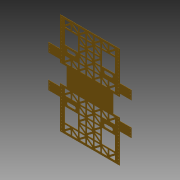
# Autodesk Inventor part: Top Plate
Saved by Autodesk Inventor 2014 SP1 (Build 180222100, 222)
## iProperties
Created: 2014-01-19
Part Number: Top Plate
Material: Aluminum 6061
Document SubType Name: Sheet Metal
Designer: Nick
Density: 2.71 g/cm^3
Appearance: Brass - Satin
Mass: 1865.48 g
Surface Area: 6483.38 cm^2
Volume: 688.368 cm^3
Sheet Metal Rule: Default
Author: Nick
Autodesk Inventor part; units mm, degrees
(part 1 of 3)
ref_plane "YZ Plane" through (0, 0, 0) normal (1, 0, 0) x (0, 1, 0)
ref_plane "XZ Plane" through (0, 0, 0) normal (0, 1, 0) x (-1, 0, 0)
ref_plane "XY Plane" through (0, 0, 0) normal (0, 0, 1) x (1, 0, 0)
sketch "Sketch1" plane through (0, 0, 0) normal (0, 0, 1) x (1, 0, 0)
  line L0 (-228.6, 152.4) -> (-228.6, 406.4)
  line L1 (-228.6, 406.4) -> (279.4, 406.4)
  line L2 (279.4, 406.4) -> (279.4, 152.4)
  line L3 (279.4, 152.4) -> (381, 152.4)
  line L4 (381, 152.4) -> (381, 76.2)
  line L5 (381, 76.2) -> (279.4, 76.2)
  line L6 (279.4, 76.2) -> (279.4, -127)
  line L7 (279.4, -127) -> (381, -127)
  line L8 (381, -127) -> (381, -203.2)
  line L9 (381, -203.2) -> (279.4, -203.2)
  line L10 (279.4, -203.2) -> (279.4, -457.2)
  line L11 (279.4, -457.2) -> (-228.6, -457.2)
  line L12 (-228.6, -457.2) -> (-228.6, -203.2)
  line L13 (-228.6, -203.2) -> (-330.2, -203.2)
  line L14 (-330.2, -203.2) -> (-330.2, -127)
  line L15 (-330.2, -127) -> (-228.6, -127)
  line L16 (-228.6, -127) -> (-228.6, 76.2)
  line L17 (-228.6, 76.2) -> (-330.2, 76.2)
  line L18 (-330.2, 76.2) -> (-330.2, 152.4)
  line L19 (-330.2, 152.4) -> (-228.6, 152.4)
  point P0 (0, 0)
  point P1 (279.4, 279.4)
  point P2 (279.4, -25.4)
  point P3 (279.4, -330.2)
  point P4 (381, -165.1)
  point P5 (381, 114.3)
  point P6 (-228.6, 279.4)
  point P7 (-228.6, -25.4)
  point P8 (-228.6, -330.2)
  point P9 (-330.2, -165.1)
  point P10 (-330.2, 114.3)
  point P11 (330.2, 76.2)
  point P12 (-279.4, 76.2)
  point P13 (-279.4, 152.4)
  point P14 (330.2, 152.4)
  point P15 (330.2, -127)
  point P16 (-279.4, -127)
  point P17 (-279.4, -203.2)
  point P18 (330.2, -203.2)
  dimension "d0" = 101.6
  dimension "d1" = 508
  dimension "d2" = 254
  dimension "d3" = 76.2
  dimension "d4" = 203.2
  dimension "d96" = 457.2
  dimension "d97" = 279.4
  constraints: 40 end point, 18 midpoint, 9 perpendicular, 6 horizontal, 6 vertical alignment, 5 collinear, 4 horizontal alignment, 2 parallel, 1 vertical
  measures "d0" distance from line of point (381, 114.3) L2
  measures "d1" distance of L0.end L1.end
  measures "d2" distance of L1.end L2.end
  measures "d3" distance of L3.end L4.end
  measures "d4" distance of L5.end L6.end
  measures "d96" distance from line of point (0, 0) L11
  measures "d97" distance from line of L6 point (0, 0)
extrude "Extrusion1" add sketch "Sketch1" along normal blind 2.286
sketch "Sketch2" plane through (0, 0, 2.286) normal (0, 0, 1) x (1, 0, 0)
  line L0 (-228.6, 406.4) -> (279.4, 406.4) projected
  line L1 (-228.6, 152.4) -> (-228.6, 406.4) projected
  line L2 (-330.2, 76.2) -> (-330.2, 152.4) projected
  line L3 (381, 152.4) -> (381, 76.2) projected
  line L4 (279.4, 406.4) -> (279.4, 152.4) projected
  point P0 (0, 0)
  point P1 (-215.9, 393.7)
  point P2 (266.7, 393.7)
  point P3 (-215.9, 368.3)
  point P4 (266.7, 368.3)
  point P5 (-215.9, 342.9)
  point P6 (266.7, 342.9)
  point P7 (-215.9, 317.5)
  point P8 (266.7, 317.5)
  point P9 (-215.9, 292.1)
  point P10 (266.7, 292.1)
  point P11 (-215.9, 266.7)
  point P12 (266.7, 266.7)
  point P13 (-215.9, 241.3)
  point P14 (266.7, 241.3)
  point P15 (-215.9, 215.9)
  point P16 (266.7, 215.9)
  point P17 (-215.9, 190.5)
  point P18 (266.7, 190.5)
  point P19 (-215.9, 165.1)
  point P20 (266.7, 165.1)
  point P21 (-215.9, 139.7)
  point P22 (266.7, 139.7)
  point P23 (-215.9, 114.3)
  point P24 (266.7, 114.3)
  point P25 (-215.9, 88.9)
  point P26 (266.7, 88.9)
  point P27 (-215.9, 63.5)
  point P28 (266.7, 63.5)
  point P29 (-215.9, 38.1)
  point P30 (266.7, 38.1)
  point P31 (-215.9, 12.7)
  point P32 (266.7, 12.7)
  point P33 (-215.9, -12.7)
  point P34 (266.7, -12.7)
  point P35 (-215.9, -38.1)
  point P36 (266.7, -38.1)
  point P37 (-215.9, -63.5)
  point P38 (266.7, -63.5)
  point P39 (-215.9, -88.9)
  point P40 (266.7, -88.9)
  point P41 (-215.9, -114.3)
  point P42 (266.7, -114.3)
  point P43 (-215.9, -139.7)
  point P44 (266.7, -139.7)
  point P45 (-215.9, -165.1)
  point P46 (266.7, -165.1)
  point P47 (-215.9, -190.5)
  point P48 (266.7, -190.5)
  point P49 (-215.9, -215.9)
  point P50 (266.7, -215.9)
  point P51 (-215.9, -241.3)
  point P52 (266.7, -241.3)
  point P53 (-215.9, -266.7)
  point P54 (266.7, -266.7)
  point P55 (-215.9, -292.1)
  point P56 (266.7, -292.1)
  point P57 (-215.9, -317.5)
  point P58 (266.7, -317.5)
  point P59 (-215.9, -342.9)
  point P60 (266.7, -342.9)
  point P61 (-215.9, -368.3)
  point P62 (266.7, -368.3)
  point P63 (-215.9, -393.7)
  point P64 (266.7, -393.7)
  point P65 (-215.9, -419.1)
  point P66 (266.7, -419.1)
  point P67 (-215.9, -444.5)
  point P68 (266.7, -444.5)
  point P69 (-317.5, 139.7)
  point P70 (-317.5, 114.3)
  point P71 (-317.5, 88.9)
  point P72 (-317.5, -139.7)
  point P73 (-317.5, -165.1)
  point P74 (-317.5, -190.5)
  point P75 (368.3, -139.7)
  point P76 (368.3, -165.1)
  point P77 (368.3, -190.5)
  point P78 (368.3, 139.7)
  point P79 (368.3, 114.3)
  point P80 (368.3, 88.9)
  dimension "d7" = 12.7
  dimension "d8" = 12.7
  dimension "d9" = 12.7
  dimension "d10" = 12.7
  dimension "d13" = 25.4
  dimension "d18" = 12.7
  dimension "d19" = 12.7
  constraints: 12 horizontal alignment, 10 vertical alignment, 1 vertical, 66 other
  measures "d7" distance from line of point (-215.9, 393.7) L1
  measures "d8" distance from line of L0 point (-215.9, 393.7)
  measures "d9" distance from line of L0 point (266.7, 393.7)
  measures "d10" distance from line of L4 point (266.7, 393.7)
  measures "d13" distance of point (-215.9, 393.7) point (-215.9, 368.3)
  measures "d18" distance from line of L3 point (368.3, 114.3)
  measures "d19" distance from line of L2 point (-317.5, 139.7)
hole "Hole1" at (-215.9, 393.7, 2.286) at (266.7, 393.7, 2.286) at (-215.9, 368.3, 2.286) at (266.7, 368.3, 2.286) at (-215.9, 342.9, 2.286) at (266.7, 342.9, 2.286) at (-215.9, 317.5, 2.286) at (266.7, 317.5, 2.286) at (-215.9, 292.1, 2.286) at (266.7, 292.1, 2.286) at (-215.9, 266.7, 2.286) at (266.7, 266.7, 2.286) at (-215.9, 241.3, 2.286) at (266.7, 241.3, 2.286) at (-215.9, 215.9, 2.286) at (266.7, 215.9, 2.286) at (-215.9, 190.5, 2.286) at (266.7, 190.5, 2.286) at (-215.9, 165.1, 2.286) at (266.7, 165.1, 2.286) at (-215.9, 139.7, 2.286) at (266.7, 139.7, 2.286) at (-215.9, 114.3, 2.286) at (266.7, 114.3, 2.286) at (-215.9, 88.9, 2.286) at (266.7, 88.9, 2.286) at (-215.9, 63.5, 2.286) at (266.7, 63.5, 2.286) at (-215.9, 38.1, 2.286) at (266.7, 38.1, 2.286) at (-215.9, 12.7, 2.286) at (266.7, 12.7, 2.286) at (-215.9, -12.7, 2.286) at (266.7, -12.7, 2.286) at (-215.9, -38.1, 2.286) at (266.7, -38.1, 2.286) at (-215.9, -63.5, 2.286) at (266.7, -63.5, 2.286) at (-215.9, -88.9, 2.286) at (266.7, -88.9, 2.286) at (-215.9, -114.3, 2.286) at (266.7, -114.3, 2.286) at (-215.9, -139.7, 2.286) at (266.7, -139.7, 2.286) at (-215.9, -165.1, 2.286) at (266.7, -165.1, 2.286) at (-215.9, -190.5, 2.286) at (266.7, -190.5, 2.286) at (-215.9, -215.9, 2.286) at (266.7, -215.9, 2.286) direction (0, 0, -1) diameter 6.7564 end through all and at (-215.9, -241.3, 2.286) (266.7, -241.3, 2.286) (-215.9, -266.7, 2.286) (266.7, -266.7, 2.286) (-215.9, -292.1, 2.286) (266.7, -292.1, 2.286) (-215.9, -317.5, 2.286) (266.7, -317.5, 2.286) (-215.9, -342.9, 2.286) (266.7, -342.9, 2.286) (-215.9, -368.3, 2.286) (266.7, -368.3, 2.286) (-215.9, -393.7, 2.286) (266.7, -393.7, 2.286) (-215.9, -419.1, 2.286) (266.7, -419.1, 2.286) (-215.9, -444.5, 2.286) (266.7, -444.5, 2.286) (-317.5, 139.7, 2.286) (-317.5, 114.3, 2.286) (-317.5, 88.9, 2.286) (-317.5, -139.7, 2.286) (-317.5, -165.1, 2.286) (-317.5, -190.5, 2.286) (368.3, -139.7, 2.286) (368.3, -165.1, 2.286) (368.3, -190.5, 2.286) (368.3, 139.7, 2.286) (368.3, 114.3, 2.286) (368.3, 88.9, 2.286)
sketch "Sketch4" plane through (0, 0, 2.286) normal (0, 0, 1) x (1, 0, 0)
  circle A0 centre (266.7, -88.9) radius 3.3782 projected
  circle A1 centre (-215.9, -88.9) radius 3.3782 projected
  circle A2 centre (266.7, -63.5) radius 3.3782 projected
  circle A3 centre (-215.9, -63.5) radius 3.3782 projected
  circle A4 centre (266.7, -38.1) radius 3.3782 projected
  circle A5 centre (-215.9, -38.1) radius 3.3782 projected
  circle A6 centre (266.7, -12.7) radius 3.3782 projected
  circle A7 centre (-215.9, -12.7) radius 3.3782 projected
  circle A8 centre (266.7, 12.7) radius 3.3782 projected
  circle A9 centre (-215.9, 12.7) radius 3.3782 projected
  circle A10 centre (266.7, 38.1) radius 3.3782 projected
  circle A11 centre (-215.9, 38.1) radius 3.3782 projected
  line L0 (-228.6, 76.2) -> (-330.2, 76.2) projected
  line L1 (-228.6, -127) -> (-228.6, 76.2) projected
  line L2 (279.4, 76.2) -> (279.4, -127) projected
  line L3 (381, 76.2) -> (279.4, 76.2) projected
  line L4 (-228.6, -101.6) -> (-171.45, -101.6)
  line L5 (-171.45, -101.6) -> (-171.45, 50.8)
  line L6 (-171.45, 50.8) -> (-228.6, 50.8)
  line L7 (-228.6, 50.8) -> (-228.6, -101.6)
  line L8 (279.4, -101.6) -> (222.25, -101.6)
  line L9 (222.25, -101.6) -> (222.25, 50.8)
  line L10 (222.25, 50.8) -> (279.4, 50.8)
  line L11 (279.4, 50.8) -> (279.4, -101.6)
  point P0 (0, 0)
  dimension "d27" = 152.4
  dimension "d28" = 57.15
  dimension "d29" = 57.15
  dimension "d30" = 152.4
  dimension "d31" = 25.4
  dimension "d32" = 25.4
  constraints: 16 end point, 4 parallel, 2 horizontal, 2 perpendicular, 2 point on line
  measures "d27" distance of L8.end L9.end
  measures "d28" distance of L9.end L10.end
  measures "d29" distance of L5.end L6.end
  measures "d30" distance of L4.end L5.end
  measures "d31" distance between parallel lines of L0 L6
  measures "d32" distance between parallel lines of L3 L10
extrude "Extrusion2" cut sketch "Sketch4" against normal through all
sketch "Sketch6" plane through (0, 0, 2.286) normal (0, 0, 1) x (1, 0, 0)
  line L0 (-171.45, -101.6) -> (-228.6, -101.6) projected
  line L1 (-228.6, -127) -> (-228.6, -101.6) projected
  line L2 (-330.2, -127) -> (-228.6, -127) projected
  line L3 (-330.2, -203.2) -> (-330.2, -127) projected
  line L4 (-228.6, -203.2) -> (-330.2, -203.2) projected
  line L5 (-228.6, -457.2) -> (-228.6, -203.2) projected
  line L6 (279.4, -457.2) -> (-228.6, -457.2) projected
  line L7 (279.4, -203.2) -> (279.4, -457.2) projected
  line L8 (381, -203.2) -> (279.4, -203.2) projected
  line L9 (381, -127) -> (381, -203.2) projected
  line L10 (279.4, -127) -> (381, -127) projected
  line L11 (279.4, -101.6) -> (279.4, -127) projected
  line L12 (279.4, -101.6) -> (222.25, -101.6) projected
  line L13 (222.25, -101.6) -> (222.25, 50.8) projected
  line L14 (279.4, 76.2) -> (279.4, 50.8) projected
  line L15 (381, 76.2) -> (279.4, 76.2) projected
  line L16 (381, 152.4) -> (381, 76.2) projected
  line L17 (279.4, 152.4) -> (381, 152.4) projected
  line L18 (279.4, 406.4) -> (279.4, 152.4) projected
  line L19 (-228.6, 406.4) -> (279.4, 406.4) projected
  line L20 (-228.6, 152.4) -> (-228.6, 406.4) projected
  line L21 (-330.2, 152.4) -> (-228.6, 152.4) projected
  line L22 (-330.2, 76.2) -> (-330.2, 152.4) projected
  line L23 (-228.6, 76.2) -> (-330.2, 76.2) projected
  line L24 (-228.6, 50.8) -> (-228.6, 76.2) projected
  line L25 (-171.45, 50.8) -> (-171.45, -101.6) projected
  circle A0 centre (368.3, 88.9) radius 3.3782 projected
  circle A1 centre (368.3, 114.3) radius 3.3782 projected
  circle A2 centre (368.3, 139.7) radius 3.3782 projected
  circle A3 centre (368.3, -190.5) radius 3.3782 projected
  circle A4 centre (368.3, -165.1) radius 3.3782 projected
  circle A5 centre (368.3, -139.7) radius 3.3782 projected
  circle A6 centre (-317.5, -190.5) radius 3.3782 projected
  circle A7 centre (-317.5, -165.1) radius 3.3782 projected
  circle A8 centre (-317.5, -139.7) radius 3.3782 projected
  circle A9 centre (-317.5, 88.9) radius 3.3782 projected
  circle A10 centre (-317.5, 114.3) radius 3.3782 projected
  circle A11 centre (-317.5, 139.7) radius 3.3782 projected
  circle A12 centre (266.7, -444.5) radius 3.3782 projected
  circle A13 centre (-215.9, -444.5) radius 3.3782 projected
  circle A14 centre (266.7, -419.1) radius 3.3782 projected
  circle A15 centre (-215.9, -419.1) radius 3.3782 projected
  circle A16 centre (266.7, -393.7) radius 3.3782 projected
  circle A17 centre (-215.9, -393.7) radius 3.3782 projected
  circle A18 centre (266.7, -368.3) radius 3.3782 projected
  circle A19 centre (-215.9, -368.3) radius 3.3782 projected
  circle A20 centre (266.7, -342.9) radius 3.3782 projected
  circle A21 centre (-215.9, -342.9) radius 3.3782 projected
  circle A22 centre (266.7, -317.5) radius 3.3782 projected
  circle A23 centre (-215.9, -317.5) radius 3.3782 projected
  circle A24 centre (266.7, -292.1) radius 3.3782 projected
  circle A25 centre (-215.9, -292.1) radius 3.3782 projected
  circle A26 centre (266.7, -266.7) radius 3.3782 projected
  circle A27 centre (-215.9, -266.7) radius 3.3782 projected
  circle A28 centre (266.7, -241.3) radius 3.3782 projected
  circle A29 centre (-215.9, -241.3) radius 3.3782 projected
  circle A30 centre (266.7, -215.9) radius 3.3782 projected
  circle A31 centre (-215.9, -215.9) radius 3.3782 projected
  circle A32 centre (266.7, -190.5) radius 3.3782 projected
  circle A33 centre (-215.9, -190.5) radius 3.3782 projected
  circle A34 centre (266.7, -165.1) radius 3.3782 projected
  circle A35 centre (-215.9, -165.1) radius 3.3782 projected
  circle A36 centre (266.7, -139.7) radius 3.3782 projected
  circle A37 centre (-215.9, -139.7) radius 3.3782 projected
  circle A38 centre (266.7, -114.3) radius 3.3782 projected
  circle A39 centre (-215.9, -114.3) radius 3.3782 projected
  line L26 (-190.5, 385.7625) -> (-190.5, 357.1875)
  line L27 (-185.42, 354.6475) -> (-147.32, 383.2225)
  line L28 (-149.225, 388.9375) -> (-187.325, 388.9375)
  line L29 (-182.88, 340.6775) -> (-144.78, 369.2525)
  line L30 (-139.7, 366.7125) -> (-139.7, 338.1375)
  line L31 (-142.875, 334.9625) -> (-180.975, 334.9625)
  arc A40 (-190.5, 357.1875) -> (-185.42, 354.6475) centre (-187.325, 357.1875) ccw
  arc A41 (-187.325, 388.9375) -> (-190.5, 385.7625) centre (-187.325, 385.7625) ccw
  arc A42 (-147.32, 383.2225) -> (-149.225, 388.9375) centre (-149.225, 385.7625) ccw
  arc A43 (-139.7, 366.7125) -> (-144.78, 369.2525) centre (-142.875, 366.7125) ccw
  arc A44 (-142.875, 334.9625) -> (-139.7, 338.1375) centre (-142.875, 338.1375) ccw
  arc A45 (-182.88, 340.6775) -> (-180.975, 334.9625) centre (-180.975, 338.1375) ccw
  line L32 (-133.35, 390.3218) -> (-133.35, 314.1218) construction
  line L33 (-76.2, 385.7625) -> (-76.2, 357.1875)
  line L34 (-81.28, 354.6475) -> (-119.38, 383.2225)
  line L35 (-117.475, 388.9375) -> (-79.375, 388.9375)
  line L36 (-83.82, 340.6775) -> (-121.92, 369.2525)
  line L37 (-127, 366.7125) -> (-127, 338.1375)
  line L38 (-123.825, 334.9625) -> (-85.725, 334.9625)
  arc A46 (-81.28, 354.6475) -> (-76.2, 357.1875) centre (-79.375, 357.1875) ccw
  arc A47 (-76.2, 385.7625) -> (-79.375, 388.9375) centre (-79.375, 385.7625) ccw
  arc A48 (-117.475, 388.9375) -> (-119.38, 383.2225) centre (-117.475, 385.7625) ccw
  arc A49 (-121.92, 369.2525) -> (-127, 366.7125) centre (-123.825, 366.7125) ccw
  arc A50 (-127, 338.1375) -> (-123.825, 334.9625) centre (-123.825, 338.1375) ccw
  arc A51 (-85.725, 334.9625) -> (-83.82, 340.6775) centre (-85.725, 338.1375) ccw
  line L39 (-192.1848, 328.6125) -> (-47.7209, 328.6125) construction
  line L40 (-190.5, 271.4625) -> (-190.5, 300.0375)
  line L41 (-185.42, 302.5775) -> (-147.32, 274.0025)
  line L42 (-149.225, 268.2875) -> (-187.325, 268.2875)
  line L43 (-182.88, 316.5475) -> (-144.78, 287.9725)
  line L44 (-139.7, 290.5125) -> (-139.7, 319.0875)
  line L45 (-142.875, 322.2625) -> (-180.975, 322.2625)
  arc A52 (-185.42, 302.5775) -> (-190.5, 300.0375) centre (-187.325, 300.0375) ccw
  arc A53 (-190.5, 271.4625) -> (-187.325, 268.2875) centre (-187.325, 271.4625) ccw
  arc A54 (-149.225, 268.2875) -> (-147.32, 274.0025) centre (-149.225, 271.4625) ccw
  arc A55 (-144.78, 287.9725) -> (-139.7, 290.5125) centre (-142.875, 290.5125) ccw
  arc A56 (-139.7, 319.0875) -> (-142.875, 322.2625) centre (-142.875, 319.0875) ccw
  arc A57 (-180.975, 322.2625) -> (-182.88, 316.5475) centre (-180.975, 319.0875) ccw
  line L46 (-127, 290.5125) -> (-127, 319.0875)
  arc A58 (-127, 290.5125) -> (-121.92, 287.9725) centre (-123.825, 290.5125) ccw
  arc A59 (-119.38, 274.0025) -> (-117.475, 268.2875) centre (-117.475, 271.4625) ccw
  line L47 (-76.2, 271.4625) -> (-76.2, 300.0375)
  arc A60 (-79.375, 268.2875) -> (-76.2, 271.4625) centre (-79.375, 271.4625) ccw
  line L48 (-117.475, 268.2875) -> (-79.375, 268.2875)
  arc A61 (-83.82, 316.5475) -> (-85.725, 322.2625) centre (-85.725, 319.0875) ccw
  line L49 (-81.28, 302.5775) -> (-119.38, 274.0025)
  line L50 (-83.82, 316.5475) -> (-121.92, 287.9725)
  line L51 (-123.825, 322.2625) -> (-85.725, 322.2625)
  arc A62 (-76.2, 300.0375) -> (-81.28, 302.5775) centre (-79.375, 300.0375) ccw
  arc A63 (-123.825, 322.2625) -> (-127, 319.0875) centre (-123.825, 319.0875) ccw
  line L52 (-63.5, 385.7625) -> (-63.5, 357.1875)
  line L53 (-58.42, 354.6475) -> (-20.32, 383.2225)
  line L54 (-22.225, 388.9375) -> (-60.325, 388.9375)
  line L55 (-55.88, 340.6775) -> (-17.78, 369.2525)
  line L56 (-12.7, 366.7125) -> (-12.7, 338.1375)
  line L57 (-15.875, 334.9625) -> (-53.975, 334.9625)
  arc A64 (-63.5, 357.1875) -> (-58.42, 354.6475) centre (-60.325, 357.1875) ccw
  arc A65 (-60.325, 388.9375) -> (-63.5, 385.7625) centre (-60.325, 385.7625) ccw
  arc A66 (-20.32, 383.2225) -> (-22.225, 388.9375) centre (-22.225, 385.7625) ccw
  arc A67 (-12.7, 366.7125) -> (-17.78, 369.2525) centre (-15.875, 366.7125) ccw
  arc A68 (-15.875, 334.9625) -> (-12.7, 338.1375) centre (-15.875, 338.1375) ccw
  arc A69 (-55.88, 340.6775) -> (-53.975, 334.9625) centre (-53.975, 338.1375) ccw
  line L58 (-6.35, 391.9093) -> (-6.35, 315.7093) construction
  line L59 (0, 366.7125) -> (0, 338.1375)
  arc A70 (5.08, 369.2525) -> (0, 366.7125) centre (3.175, 366.7125) ccw
  arc A71 (9.525, 388.9375) -> (7.62, 383.2225) centre (9.525, 385.7625) ccw
  line L60 (50.8, 385.7625) -> (50.8, 357.1875)
  arc A72 (50.8, 385.7625) -> (47.625, 388.9375) centre (47.625, 385.7625) ccw
  line L61 (9.525, 388.9375) -> (47.625, 388.9375)
  arc A73 (41.275, 334.9625) -> (43.18, 340.6775) centre (41.275, 338.1375) ccw
  line L62 (45.72, 354.6475) -> (7.62, 383.2225)
  line L63 (43.18, 340.6775) -> (5.08, 369.2525)
  line L64 (3.175, 334.9625) -> (41.275, 334.9625)
  arc A74 (45.72, 354.6475) -> (50.8, 357.1875) centre (47.625, 357.1875) ccw
  arc A75 (0, 338.1375) -> (3.175, 334.9625) centre (3.175, 338.1375) ccw
  line L65 (-190.5973, 328.6125) -> (-46.1334, 328.6125) construction
  line L66 (0, 290.5125) -> (0, 319.0875)
  arc A76 (-53.975, 322.2625) -> (-55.88, 316.5475) centre (-53.975, 319.0875) ccw
  line L67 (-15.875, 322.2625) -> (-53.975, 322.2625)
  arc A77 (-12.7, 319.0875) -> (-15.875, 322.2625) centre (-15.875, 319.0875) ccw
  line L68 (-63.5, 271.4625) -> (-63.5, 300.0375)
  line L69 (-55.88, 316.5475) -> (-17.78, 287.9725)
  line L70 (-12.7, 290.5125) -> (-12.7, 319.0875)
  line L71 (-58.42, 302.5775) -> (-20.32, 274.0025)
  arc A78 (-22.225, 268.2875) -> (-20.32, 274.0025) centre (-22.225, 271.4625) ccw
  line L72 (-22.225, 268.2875) -> (-60.325, 268.2875)
  arc A79 (-17.78, 287.9725) -> (-12.7, 290.5125) centre (-15.875, 290.5125) ccw
  line L73 (50.8, 271.4625) -> (50.8, 300.0375)
  arc A80 (-58.42, 302.5775) -> (-63.5, 300.0375) centre (-60.325, 300.0375) ccw
  arc A81 (3.175, 322.2625) -> (0, 319.0875) centre (3.175, 319.0875) ccw
  arc A82 (0, 290.5125) -> (5.08, 287.9725) centre (3.175, 290.5125) ccw
  arc A83 (-63.5, 271.4625) -> (-60.325, 268.2875) centre (-60.325, 271.4625) ccw
  line L74 (3.175, 322.2625) -> (41.275, 322.2625)
  line L75 (43.18, 316.5475) -> (5.08, 287.9725)
  arc A84 (43.18, 316.5475) -> (41.275, 322.2625) centre (41.275, 319.0875) ccw
  arc A85 (50.8, 300.0375) -> (45.72, 302.5775) centre (47.625, 300.0375) ccw
  arc A86 (7.62, 274.0025) -> (9.525, 268.2875) centre (9.525, 271.4625) ccw
  line L76 (9.525, 268.2875) -> (47.625, 268.2875)
  arc A87 (47.625, 268.2875) -> (50.8, 271.4625) centre (47.625, 271.4625) ccw
  line L77 (45.72, 302.5775) -> (7.62, 274.0025)
  line L78 (63.5, 385.7625) -> (63.5, 357.1875)
  line L79 (68.58, 354.6475) -> (106.68, 383.2225)
  line L80 (104.775, 388.9375) -> (66.675, 388.9375)
  line L81 (71.12, 340.6775) -> (109.22, 369.2525)
  line L82 (114.3, 366.7125) -> (114.3, 338.1375)
  line L83 (111.125, 334.9625) -> (73.025, 334.9625)
  arc A88 (63.5, 357.1875) -> (68.58, 354.6475) centre (66.675, 357.1875) ccw
  arc A89 (66.675, 388.9375) -> (63.5, 385.7625) centre (66.675, 385.7625) ccw
  arc A90 (106.68, 383.2225) -> (104.775, 388.9375) centre (104.775, 385.7625) ccw
  arc A91 (114.3, 366.7125) -> (109.22, 369.2525) centre (111.125, 366.7125) ccw
  arc A92 (111.125, 334.9625) -> (114.3, 338.1375) centre (111.125, 338.1375) ccw
  arc A93 (71.12, 340.6775) -> (73.025, 334.9625) centre (73.025, 338.1375) ccw
  line L84 (120.65, 391.9093) -> (120.65, 315.7093) construction
  line L85 (127, 366.7125) -> (127, 338.1375)
  arc A94 (132.08, 369.2525) -> (127, 366.7125) centre (130.175, 366.7125) ccw
  arc A95 (136.525, 388.9375) -> (134.62, 383.2225) centre (136.525, 385.7625) ccw
  line L86 (177.8, 385.7625) -> (177.8, 357.1875)
  arc A96 (177.8, 385.7625) -> (174.625, 388.9375) centre (174.625, 385.7625) ccw
  line L87 (136.525, 388.9375) -> (174.625, 388.9375)
  arc A97 (168.275, 334.9625) -> (170.18, 340.6775) centre (168.275, 338.1375) ccw
  line L88 (172.72, 354.6475) -> (134.62, 383.2225)
  line L89 (170.18, 340.6775) -> (132.08, 369.2525)
  line L90 (130.175, 334.9625) -> (168.275, 334.9625)
  arc A98 (172.72, 354.6475) -> (177.8, 357.1875) centre (174.625, 357.1875) ccw
  arc A99 (127, 338.1375) -> (130.175, 334.9625) centre (130.175, 338.1375) ccw
  line L91 (-190.5973, 328.6125) -> (-46.1334, 328.6125) construction
  line L92 (127, 290.5125) -> (127, 319.0875)
  arc A100 (73.025, 322.2625) -> (71.12, 316.5475) centre (73.025, 319.0875) ccw
  line L93 (111.125, 322.2625) -> (73.025, 322.2625)
  arc A101 (114.3, 319.0875) -> (111.125, 322.2625) centre (111.125, 319.0875) ccw
  line L94 (63.5, 271.4625) -> (63.5, 300.0375)
  line L95 (71.12, 316.5475) -> (109.22, 287.9725)
  line L96 (114.3, 290.5125) -> (114.3, 319.0875)
  line L97 (68.58, 302.5775) -> (106.68, 274.0025)
  arc A102 (104.775, 268.2875) -> (106.68, 274.0025) centre (104.775, 271.4625) ccw
  line L98 (104.775, 268.2875) -> (66.675, 268.2875)
  arc A103 (109.22, 287.9725) -> (114.3, 290.5125) centre (111.125, 290.5125) ccw
  line L99 (177.8, 271.4625) -> (177.8, 300.0375)
  arc A104 (68.58, 302.5775) -> (63.5, 300.0375) centre (66.675, 300.0375) ccw
  arc A105 (130.175, 322.2625) -> (127, 319.0875) centre (130.175, 319.0875) ccw
  arc A106 (127, 290.5125) -> (132.08, 287.9725) centre (130.175, 290.5125) ccw
  arc A107 (63.5, 271.4625) -> (66.675, 268.2875) centre (66.675, 271.4625) ccw
  line L100 (130.175, 322.2625) -> (168.275, 322.2625)
  line L101 (170.18, 316.5475) -> (132.08, 287.9725)
  arc A108 (170.18, 316.5475) -> (168.275, 322.2625) centre (168.275, 319.0875) ccw
  arc A109 (177.8, 300.0375) -> (172.72, 302.5775) centre (174.625, 300.0375) ccw
  arc A110 (134.62, 274.0025) -> (136.525, 268.2875) centre (136.525, 271.4625) ccw
  line L102 (136.525, 268.2875) -> (174.625, 268.2875)
  arc A111 (174.625, 268.2875) -> (177.8, 271.4625) centre (174.625, 271.4625) ccw
  line L103 (172.72, 302.5775) -> (134.62, 274.0025)
  line L104 (190.5, 385.7625) -> (190.5, 357.1875)
  arc A112 (193.675, 388.9375) -> (190.5, 385.7625) centre (193.675, 385.7625) ccw
  line L105 (195.58, 354.6475) -> (233.68, 383.2225)
  line L106 (231.775, 388.9375) -> (193.675, 388.9375)
  arc A113 (233.68, 383.2225) -> (231.775, 388.9375) centre (231.775, 385.7625) ccw
  arc A114 (241.3, 366.7125) -> (236.22, 369.2525) centre (238.125, 366.7125) ccw
  line L107 (198.12, 340.6775) -> (236.22, 369.2525)
  line L108 (241.3, 366.7125) -> (241.3, 338.1375)
  line L109 (238.125, 334.9625) -> (200.025, 334.9625)
  arc A115 (190.5, 357.1875) -> (195.58, 354.6475) centre (193.675, 357.1875) ccw
  arc A116 (198.12, 340.6775) -> (200.025, 334.9625) centre (200.025, 338.1375) ccw
  arc A117 (238.125, 334.9625) -> (241.3, 338.1375) centre (238.125, 338.1375) ccw
  line L110 (241.3, 290.5125) -> (241.3, 319.0875)
  line L111 (-189.0098, 328.6125) -> (-44.5459, 328.6125) construction
  arc A118 (241.3, 319.0875) -> (238.125, 322.2625) centre (238.125, 319.0875) ccw
  arc A119 (236.22, 287.9725) -> (241.3, 290.5125) centre (238.125, 290.5125) ccw
  arc A120 (190.5, 271.4625) -> (193.675, 268.2875) centre (193.675, 271.4625) ccw
  line L112 (190.5, 271.4625) -> (190.5, 300.0375)
  line L113 (231.775, 268.2875) -> (193.675, 268.2875)
  arc A121 (195.58, 302.5775) -> (190.5, 300.0375) centre (193.675, 300.0375) ccw
  arc A122 (231.775, 268.2875) -> (233.68, 274.0025) centre (231.775, 271.4625) ccw
  arc A123 (200.025, 322.2625) -> (198.12, 316.5475) centre (200.025, 319.0875) ccw
  line L114 (195.58, 302.5775) -> (233.68, 274.0025)
  line L115 (198.12, 316.5475) -> (236.22, 287.9725)
  line L116 (238.125, 322.2625) -> (200.025, 322.2625)
  line L117 (-190.5, 252.4125) -> (-190.5, 223.8375)
  line L118 (-185.42, 221.2975) -> (-147.32, 249.8725)
  line L119 (-149.225, 255.5875) -> (-187.325, 255.5875)
  line L120 (-182.88, 207.3275) -> (-144.78, 235.9025)
  line L121 (-139.7, 233.3625) -> (-139.7, 204.7875)
  line L122 (-142.875, 201.6125) -> (-180.975, 201.6125)
  arc A124 (-190.5, 223.8375) -> (-185.42, 221.2975) centre (-187.325, 223.8375) ccw
  arc A125 (-187.325, 255.5875) -> (-190.5, 252.4125) centre (-187.325, 252.4125) ccw
  arc A126 (-147.32, 249.8725) -> (-149.225, 255.5875) centre (-149.225, 252.4125) ccw
  arc A127 (-139.7, 233.3625) -> (-144.78, 235.9025) centre (-142.875, 233.3625) ccw
  arc A128 (-142.875, 201.6125) -> (-139.7, 204.7875) centre (-142.875, 204.7875) ccw
  arc A129 (-182.88, 207.3275) -> (-180.975, 201.6125) centre (-180.975, 204.7875) ccw
  line L123 (-133.35, 391.9093) -> (-133.35, 315.7093) construction
  line L124 (-127, 233.3625) -> (-127, 204.7875)
  arc A130 (-121.92, 235.9025) -> (-127, 233.3625) centre (-123.825, 233.3625) ccw
  arc A131 (-117.475, 255.5875) -> (-119.38, 249.8725) centre (-117.475, 252.4125) ccw
  line L125 (-76.2, 252.4125) -> (-76.2, 223.8375)
  arc A132 (-76.2, 252.4125) -> (-79.375, 255.5875) centre (-79.375, 252.4125) ccw
  line L126 (-117.475, 255.5875) -> (-79.375, 255.5875)
  arc A133 (-85.725, 201.6125) -> (-83.82, 207.3275) centre (-85.725, 204.7875) ccw
  line L127 (-81.28, 221.2975) -> (-119.38, 249.8725)
  line L128 (-83.82, 207.3275) -> (-121.92, 235.9025)
  line L129 (-123.825, 201.6125) -> (-85.725, 201.6125)
  arc A134 (-81.28, 221.2975) -> (-76.2, 223.8375) centre (-79.375, 223.8375) ccw
  arc A135 (-127, 204.7875) -> (-123.825, 201.6125) centre (-123.825, 204.7875) ccw
  line L130 (-190.5973, 195.2625) -> (-46.1334, 195.2625) construction
  line L131 (-127, 157.1625) -> (-127, 185.7375)
  arc A136 (-180.975, 188.9125) -> (-182.88, 183.1975) centre (-180.975, 185.7375) ccw
  line L132 (-142.875, 188.9125) -> (-180.975, 188.9125)
  arc A137 (-139.7, 185.7375) -> (-142.875, 188.9125) centre (-142.875, 185.7375) ccw
  line L133 (-190.5, 138.1125) -> (-190.5, 166.6875)
  line L134 (-182.88, 183.1975) -> (-144.78, 154.6225)
  line L135 (-139.7, 157.1625) -> (-139.7, 185.7375)
  line L136 (-185.42, 169.2275) -> (-147.32, 140.6525)
  arc A138 (-149.225, 134.9375) -> (-147.32, 140.6525) centre (-149.225, 138.1125) ccw
  line L137 (-149.225, 134.9375) -> (-187.325, 134.9375)
  arc A139 (-144.78, 154.6225) -> (-139.7, 157.1625) centre (-142.875, 157.1625) ccw
  line L138 (-76.2, 138.1125) -> (-76.2, 166.6875)
  arc A140 (-185.42, 169.2275) -> (-190.5, 166.6875) centre (-187.325, 166.6875) ccw
  arc A141 (-123.825, 188.9125) -> (-127, 185.7375) centre (-123.825, 185.7375) ccw
  arc A142 (-127, 157.1625) -> (-121.92, 154.6225) centre (-123.825, 157.1625) ccw
  arc A143 (-190.5, 138.1125) -> (-187.325, 134.9375) centre (-187.325, 138.1125) ccw
  line L139 (-123.825, 188.9125) -> (-85.725, 188.9125)
  line L140 (-83.82, 183.1975) -> (-121.92, 154.6225)
  arc A144 (-83.82, 183.1975) -> (-85.725, 188.9125) centre (-85.725, 185.7375) ccw
  arc A145 (-76.2, 166.6875) -> (-81.28, 169.2275) centre (-79.375, 166.6875) ccw
  arc A146 (-119.38, 140.6525) -> (-117.475, 134.9375) centre (-117.475, 138.1125) ccw
  line L141 (-117.475, 134.9375) -> (-79.375, 134.9375)
  arc A147 (-79.375, 134.9375) -> (-76.2, 138.1125) centre (-79.375, 138.1125) ccw
  line L142 (-81.28, 169.2275) -> (-119.38, 140.6525)
  line L143 (-63.5, 252.4125) -> (-63.5, 223.8375)
  arc A148 (-60.325, 255.5875) -> (-63.5, 252.4125) centre (-60.325, 252.4125) ccw
  line L144 (-58.42, 221.2975) -> (-20.32, 249.8725)
  line L145 (-22.225, 255.5875) -> (-60.325, 255.5875)
  arc A149 (-20.32, 249.8725) -> (-22.225, 255.5875) centre (-22.225, 252.4125) ccw
  arc A150 (-12.7, 233.3625) -> (-17.78, 235.9025) centre (-15.875, 233.3625) ccw
  line L146 (-55.88, 207.3275) -> (-17.78, 235.9025)
  line L147 (-12.7, 233.3625) -> (-12.7, 204.7875)
  line L148 (-15.875, 201.6125) -> (-53.975, 201.6125)
  arc A151 (-63.5, 223.8375) -> (-58.42, 221.2975) centre (-60.325, 223.8375) ccw
  arc A152 (-55.88, 207.3275) -> (-53.975, 201.6125) centre (-53.975, 204.7875) ccw
  arc A153 (-15.875, 201.6125) -> (-12.7, 204.7875) centre (-15.875, 204.7875) ccw
  arc A154 (47.625, 134.9375) -> (50.8, 138.1125) centre (47.625, 138.1125) ccw
  arc A155 (43.18, 183.1975) -> (41.275, 188.9125) centre (41.275, 185.7375) ccw
  arc A156 (3.175, 188.9125) -> (0, 185.7375) centre (3.175, 185.7375) ccw
  line L149 (-12.7, 157.1625) -> (-12.7, 185.7375)
  line L150 (-189.0098, 195.2625) -> (-44.5459, 195.2625) construction
  line L151 (0, 157.1625) -> (0, 185.7375)
  line L152 (3.175, 201.6125) -> (41.275, 201.6125)
  line L153 (3.175, 188.9125) -> (41.275, 188.9125)
  line L154 (43.18, 183.1975) -> (5.08, 154.6225)
  arc A157 (50.8, 166.6875) -> (45.72, 169.2275) centre (47.625, 166.6875) ccw
  line L155 (45.72, 169.2275) -> (7.62, 140.6525)
  line L156 (50.8, 138.1125) -> (50.8, 166.6875)
  line L157 (9.525, 134.9375) -> (47.625, 134.9375)
  arc A158 (5.08, 235.9025) -> (0, 233.3625) centre (3.175, 233.3625) ccw
  arc A159 (9.525, 255.5875) -> (7.62, 249.8725) centre (9.525, 252.4125) ccw
  line L158 (0, 233.3625) -> (0, 204.7875)
  line L159 (-6.35, 393.4968) -> (-6.35, 317.2968) construction
  arc A160 (41.275, 201.6125) -> (43.18, 207.3275) centre (41.275, 204.7875) ccw
  line L160 (43.18, 207.3275) -> (5.08, 235.9025)
  line L161 (9.525, 255.5875) -> (47.625, 255.5875)
  line L162 (45.72, 221.2975) -> (7.62, 249.8725)
  arc A161 (50.8, 252.4125) -> (47.625, 255.5875) centre (47.625, 252.4125) ccw
  line L163 (50.8, 252.4125) -> (50.8, 223.8375)
  arc A162 (45.72, 221.2975) -> (50.8, 223.8375) centre (47.625, 223.8375) ccw
  arc A163 (0, 204.7875) -> (3.175, 201.6125) centre (3.175, 204.7875) ccw
  arc A164 (-12.7, 185.7375) -> (-15.875, 188.9125) centre (-15.875, 185.7375) ccw
  arc A165 (0, 157.1625) -> (5.08, 154.6225) centre (3.175, 157.1625) ccw
  arc A166 (7.62, 140.6525) -> (9.525, 134.9375) centre (9.525, 138.1125) ccw
  arc A167 (-17.78, 154.6225) -> (-12.7, 157.1625) centre (-15.875, 157.1625) ccw
  arc A168 (-63.5, 138.1125) -> (-60.325, 134.9375) centre (-60.325, 138.1125) ccw
  line L164 (-63.5, 138.1125) -> (-63.5, 166.6875)
  line L165 (-22.225, 134.9375) -> (-60.325, 134.9375)
  arc A169 (-58.42, 169.2275) -> (-63.5, 166.6875) centre (-60.325, 166.6875) ccw
  arc A170 (-22.225, 134.9375) -> (-20.32, 140.6525) centre (-22.225, 138.1125) ccw
  arc A171 (-53.975, 188.9125) -> (-55.88, 183.1975) centre (-53.975, 185.7375) ccw
  line L166 (-58.42, 169.2275) -> (-20.32, 140.6525)
  line L167 (-55.88, 183.1975) -> (-17.78, 154.6225)
  line L168 (-15.875, 188.9125) -> (-53.975, 188.9125)
  arc A172 (66.675, 255.5875) -> (63.5, 252.4125) centre (66.675, 252.4125) ccw
  line L169 (104.775, 255.5875) -> (66.675, 255.5875)
  line L170 (127, 233.3625) -> (127, 204.7875)
  arc A173 (127, 204.7875) -> (130.175, 201.6125) centre (130.175, 204.7875) ccw
  arc A174 (132.08, 235.9025) -> (127, 233.3625) centre (130.175, 233.3625) ccw
  arc A175 (136.525, 255.5875) -> (134.62, 249.8725) centre (136.525, 252.4125) ccw
  line L171 (172.72, 221.2975) -> (134.62, 249.8725)
  line L172 (136.525, 255.5875) -> (174.625, 255.5875)
  line L173 (177.8, 252.4125) -> (177.8, 223.8375)
  line L174 (170.18, 207.3275) -> (132.08, 235.9025)
  line L175 (130.175, 201.6125) -> (168.275, 201.6125)
  arc A176 (168.275, 201.6125) -> (170.18, 207.3275) centre (168.275, 204.7875) ccw
  line L176 (-187.4223, 195.2625) -> (-42.9584, 195.2625) construction
  line L177 (-189.0098, 195.2625) -> (-44.5459, 195.2625) construction
  arc A177 (106.68, 249.8725) -> (104.775, 255.5875) centre (104.775, 252.4125) ccw
  line L178 (63.5, 252.4125) -> (63.5, 223.8375)
  arc A178 (63.5, 223.8375) -> (68.58, 221.2975) centre (66.675, 223.8375) ccw
  line L179 (68.58, 221.2975) -> (106.68, 249.8725)
  arc A179 (114.3, 233.3625) -> (109.22, 235.9025) centre (111.125, 233.3625) ccw
  line L180 (71.12, 207.3275) -> (109.22, 235.9025)
  line L181 (111.125, 201.6125) -> (73.025, 201.6125)
  line L182 (120.65, 393.4968) -> (120.65, 317.2968) construction
  line L183 (114.3, 233.3625) -> (114.3, 204.7875)
  arc A180 (111.125, 201.6125) -> (114.3, 204.7875) centre (111.125, 204.7875) ccw
  arc A181 (114.3, 185.7375) -> (111.125, 188.9125) centre (111.125, 185.7375) ccw
  line L184 (114.3, 157.1625) -> (114.3, 185.7375)
  line L185 (111.125, 188.9125) -> (73.025, 188.9125)
  arc A182 (73.025, 188.9125) -> (71.12, 183.1975) centre (73.025, 185.7375) ccw
  line L186 (71.12, 183.1975) -> (109.22, 154.6225)
  arc A183 (68.58, 169.2275) -> (63.5, 166.6875) centre (66.675, 166.6875) ccw
  line L187 (68.58, 169.2275) -> (106.68, 140.6525)
  line L188 (104.775, 134.9375) -> (66.675, 134.9375)
  line L189 (63.5, 138.1125) -> (63.5, 166.6875)
  arc A184 (63.5, 138.1125) -> (66.675, 134.9375) centre (66.675, 138.1125) ccw
  arc A185 (71.12, 207.3275) -> (73.025, 201.6125) centre (73.025, 204.7875) ccw
  line L190 (127, 157.1625) -> (127, 185.7375)
  arc A186 (104.775, 134.9375) -> (106.68, 140.6525) centre (104.775, 138.1125) ccw
  arc A187 (109.22, 154.6225) -> (114.3, 157.1625) centre (111.125, 157.1625) ccw
  arc A188 (177.8, 252.4125) -> (174.625, 255.5875) centre (174.625, 252.4125) ccw
  arc A189 (172.72, 221.2975) -> (177.8, 223.8375) centre (174.625, 223.8375) ccw
  arc A190 (198.12, 207.3275) -> (200.025, 201.6125) centre (200.025, 204.7875) ccw
  arc A191 (190.5, 223.8375) -> (195.58, 221.2975) centre (193.675, 223.8375) ccw
  line L191 (190.5, 252.4125) -> (190.5, 223.8375)
  arc A192 (193.675, 255.5875) -> (190.5, 252.4125) centre (193.675, 252.4125) ccw
  arc A193 (130.175, 188.9125) -> (127, 185.7375) centre (130.175, 185.7375) ccw
  arc A194 (127, 157.1625) -> (132.08, 154.6225) centre (130.175, 157.1625) ccw
  line L192 (130.175, 188.9125) -> (168.275, 188.9125)
  line L193 (177.8, 138.1125) -> (177.8, 166.6875)
  arc A195 (170.18, 183.1975) -> (168.275, 188.9125) centre (168.275, 185.7375) ccw
  line L194 (195.58, 221.2975) -> (233.68, 249.8725)
  line L195 (231.775, 255.5875) -> (193.675, 255.5875)
  arc A196 (241.3, 233.3625) -> (236.22, 235.9025) centre (238.125, 233.3625) ccw
  line L196 (198.12, 207.3275) -> (236.22, 235.9025)
  arc A197 (241.3, 185.7375) -> (238.125, 188.9125) centre (238.125, 185.7375) ccw
  arc A198 (238.125, 201.6125) -> (241.3, 204.7875) centre (238.125, 204.7875) ccw
  arc A199 (236.22, 154.6225) -> (241.3, 157.1625) centre (238.125, 157.1625) ccw
  arc A200 (231.775, 134.9375) -> (233.68, 140.6525) centre (231.775, 138.1125) ccw
  line L197 (170.18, 183.1975) -> (132.08, 154.6225)
  arc A201 (177.8, 166.6875) -> (172.72, 169.2275) centre (174.625, 166.6875) ccw
  arc A202 (174.625, 134.9375) -> (177.8, 138.1125) centre (174.625, 138.1125) ccw
  line L198 (136.525, 134.9375) -> (174.625, 134.9375)
  arc A203 (134.62, 140.6525) -> (136.525, 134.9375) centre (136.525, 138.1125) ccw
  line L199 (172.72, 169.2275) -> (134.62, 140.6525)
  line L200 (241.3, 233.3625) -> (241.3, 204.7875)
  arc A204 (233.68, 249.8725) -> (231.775, 255.5875) centre (231.775, 252.4125) ccw
  line L201 (238.125, 201.6125) -> (200.025, 201.6125)
  line L202 (241.3, 157.1625) -> (241.3, 185.7375)
  line L203 (238.125, 188.9125) -> (200.025, 188.9125)
  arc A205 (200.025, 188.9125) -> (198.12, 183.1975) centre (200.025, 185.7375) ccw
  line L204 (198.12, 183.1975) -> (236.22, 154.6225)
  arc A206 (195.58, 169.2275) -> (190.5, 166.6875) centre (193.675, 166.6875) ccw
  line L205 (195.58, 169.2275) -> (233.68, 140.6525)
  line L206 (231.775, 134.9375) -> (193.675, 134.9375)
  line L207 (190.5, 138.1125) -> (190.5, 166.6875)
  arc A207 (190.5, 138.1125) -> (193.675, 134.9375) centre (193.675, 138.1125) ccw
  line L208 (-190.5, 119.0625) -> (-190.5, 90.4875)
  line L209 (-185.42, 87.9475) -> (-147.32, 116.5225)
  line L210 (-149.225, 122.2375) -> (-187.325, 122.2375)
  line L211 (-182.88, 73.9775) -> (-144.78, 102.5525)
  line L212 (-139.7, 100.0125) -> (-139.7, 71.4375)
  line L213 (-142.875, 68.2625) -> (-180.975, 68.2625)
  arc A208 (-190.5, 90.4875) -> (-185.42, 87.9475) centre (-187.325, 90.4875) ccw
  arc A209 (-187.325, 122.2375) -> (-190.5, 119.0625) centre (-187.325, 119.0625) ccw
  arc A210 (-147.32, 116.5225) -> (-149.225, 122.2375) centre (-149.225, 119.0625) ccw
  arc A211 (-139.7, 100.0125) -> (-144.78, 102.5525) centre (-142.875, 100.0125) ccw
  arc A212 (-142.875, 68.2625) -> (-139.7, 71.4375) centre (-142.875, 71.4375) ccw
  arc A213 (-182.88, 73.9775) -> (-180.975, 68.2625) centre (-180.975, 71.4375) ccw
  line L214 (-133.35, 391.9093) -> (-133.35, 315.7093) construction
  line L215 (-127, 100.0125) -> (-127, 71.4375)
  arc A214 (-121.92, 102.5525) -> (-127, 100.0125) centre (-123.825, 100.0125) ccw
  arc A215 (-117.475, 122.2375) -> (-119.38, 116.5225) centre (-117.475, 119.0625) ccw
  line L216 (-76.2, 119.0625) -> (-76.2, 90.4875)
  arc A216 (-76.2, 119.0625) -> (-79.375, 122.2375) centre (-79.375, 119.0625) ccw
  line L217 (-117.475, 122.2375) -> (-79.375, 122.2375)
  arc A217 (-85.725, 68.2625) -> (-83.82, 73.9775) centre (-85.725, 71.4375) ccw
  line L218 (-81.28, 87.9475) -> (-119.38, 116.5225)
  line L219 (-83.82, 73.9775) -> (-121.92, 102.5525)
  line L220 (-123.825, 68.2625) -> (-85.725, 68.2625)
  arc A218 (-81.28, 87.9475) -> (-76.2, 90.4875) centre (-79.375, 90.4875) ccw
  arc A219 (-127, 71.4375) -> (-123.825, 68.2625) centre (-123.825, 71.4375) ccw
  line L221 (-63.5, 119.0625) -> (-63.5, 90.4875)
  arc A220 (-60.325, 122.2375) -> (-63.5, 119.0625) centre (-60.325, 119.0625) ccw
  line L222 (-58.42, 87.9475) -> (-20.32, 116.5225)
  line L223 (-22.225, 122.2375) -> (-60.325, 122.2375)
  arc A221 (-20.32, 116.5225) -> (-22.225, 122.2375) centre (-22.225, 119.0625) ccw
  arc A222 (-12.7, 100.0125) -> (-17.78, 102.5525) centre (-15.875, 100.0125) ccw
  line L224 (-55.88, 73.9775) -> (-17.78, 102.5525)
  line L225 (-12.7, 100.0125) -> (-12.7, 71.4375)
  line L226 (-15.875, 68.2625) -> (-53.975, 68.2625)
  arc A223 (-63.5, 90.4875) -> (-58.42, 87.9475) centre (-60.325, 90.4875) ccw
  arc A224 (-55.88, 73.9775) -> (-53.975, 68.2625) centre (-53.975, 71.4375) ccw
  arc A225 (-15.875, 68.2625) -> (-12.7, 71.4375) centre (-15.875, 71.4375) ccw
  line L227 (3.175, 68.2625) -> (41.275, 68.2625)
  arc A226 (5.08, 102.5525) -> (0, 100.0125) centre (3.175, 100.0125) ccw
  arc A227 (9.525, 122.2375) -> (7.62, 116.5225) centre (9.525, 119.0625) ccw
  line L228 (0, 100.0125) -> (0, 71.4375)
  line L229 (-6.35, 393.4968) -> (-6.35, 317.2968) construction
  arc A228 (41.275, 68.2625) -> (43.18, 73.9775) centre (41.275, 71.4375) ccw
  line L230 (43.18, 73.9775) -> (5.08, 102.5525)
  line L231 (9.525, 122.2375) -> (47.625, 122.2375)
  line L232 (45.72, 87.9475) -> (7.62, 116.5225)
  arc A229 (50.8, 119.0625) -> (47.625, 122.2375) centre (47.625, 119.0625) ccw
  line L233 (50.8, 119.0625) -> (50.8, 90.4875)
  arc A230 (45.72, 87.9475) -> (50.8, 90.4875) centre (47.625, 90.4875) ccw
  arc A231 (0, 71.4375) -> (3.175, 68.2625) centre (3.175, 71.4375) ccw
  arc A232 (66.675, 122.2375) -> (63.5, 119.0625) centre (66.675, 119.0625) ccw
  line L234 (104.775, 122.2375) -> (66.675, 122.2375)
  line L235 (127, 100.0125) -> (127, 71.4375)
  arc A233 (127, 71.4375) -> (130.175, 68.2625) centre (130.175, 71.4375) ccw
  arc A234 (132.08, 102.5525) -> (127, 100.0125) centre (130.175, 100.0125) ccw
  arc A235 (136.525, 122.2375) -> (134.62, 116.5225) centre (136.525, 119.0625) ccw
  line L236 (172.72, 87.9475) -> (134.62, 116.5225)
  line L237 (136.525, 122.2375) -> (174.625, 122.2375)
  line L238 (177.8, 119.0625) -> (177.8, 90.4875)
  line L239 (170.18, 73.9775) -> (132.08, 102.5525)
  line L240 (130.175, 68.2625) -> (168.275, 68.2625)
  arc A236 (168.275, 68.2625) -> (170.18, 73.9775) centre (168.275, 71.4375) ccw
  arc A237 (106.68, 116.5225) -> (104.775, 122.2375) centre (104.775, 119.0625) ccw
  line L241 (63.5, 119.0625) -> (63.5, 90.4875)
  arc A238 (63.5, 90.4875) -> (68.58, 87.9475) centre (66.675, 90.4875) ccw
  line L242 (68.58, 87.9475) -> (106.68, 116.5225)
  arc A239 (114.3, 100.0125) -> (109.22, 102.5525) centre (111.125, 100.0125) ccw
  line L243 (71.12, 73.9775) -> (109.22, 102.5525)
  line L244 (111.125, 68.2625) -> (73.025, 68.2625)
  line L245 (120.65, 393.4968) -> (120.65, 317.2968) construction
  line L246 (114.3, 100.0125) -> (114.3, 71.4375)
  arc A240 (111.125, 68.2625) -> (114.3, 71.4375) centre (111.125, 71.4375) ccw
  arc A241 (71.12, 73.9775) -> (73.025, 68.2625) centre (73.025, 71.4375) ccw
  arc A242 (177.8, 119.0625) -> (174.625, 122.2375) centre (174.625, 119.0625) ccw
  arc A243 (172.72, 87.9475) -> (177.8, 90.4875) centre (174.625, 90.4875) ccw
  arc A244 (198.12, 73.9775) -> (200.025, 68.2625) centre (200.025, 71.4375) ccw
  arc A245 (190.5, 90.4875) -> (195.58, 87.9475) centre (193.675, 90.4875) ccw
  line L247 (190.5, 119.0625) -> (190.5, 90.4875)
  arc A246 (193.675, 122.2375) -> (190.5, 119.0625) centre (193.675, 119.0625) ccw
  line L248 (195.58, 87.9475) -> (233.68, 116.5225)
  line L249 (231.775, 122.2375) -> (193.675, 122.2375)
  arc A247 (241.3, 100.0125) -> (236.22, 102.5525) centre (238.125, 100.0125) ccw
  line L250 (198.12, 73.9775) -> (236.22, 102.5525)
  arc A248 (238.125, 68.2625) -> (241.3, 71.4375) centre (238.125, 71.4375) ccw
  line L251 (241.3, 100.0125) -> (241.3, 71.4375)
  arc A249 (233.68, 116.5225) -> (231.775, 122.2375) centre (231.775, 119.0625) ccw
  line L252 (238.125, 68.2625) -> (200.025, 68.2625)
  line L253 (122.2375, 395.0843) -> (122.2375, 318.8843) construction
  line L254 (-4.7625, 395.0843) -> (-4.7625, 318.8843) construction
  line L255 (-131.7625, 393.4968) -> (-131.7625, 317.2968) construction
  line L256 (222.25, 50.8) -> (279.4, 50.8) projected
  line L257 (-228.6, 50.8) -> (-171.45, 50.8) projected
  line L258 (-190.5, -122.2375) -> (-190.5, -150.8125)
  line L259 (-185.42, -153.3525) -> (-147.32, -124.7775)
  line L260 (-149.225, -119.0625) -> (-187.325, -119.0625)
  line L261 (-182.88, -167.3225) -> (-144.78, -138.7475)
  line L262 (-139.7, -141.2875) -> (-139.7, -169.8625)
  line L263 (-142.875, -173.0375) -> (-180.975, -173.0375)
  arc A250 (-190.5, -150.8125) -> (-185.42, -153.3525) centre (-187.325, -150.8125) ccw
  arc A251 (-187.325, -119.0625) -> (-190.5, -122.2375) centre (-187.325, -122.2375) ccw
  arc A252 (-147.32, -124.7775) -> (-149.225, -119.0625) centre (-149.225, -122.2375) ccw
  arc A253 (-139.7, -141.2875) -> (-144.78, -138.7475) centre (-142.875, -141.2875) ccw
  arc A254 (-142.875, -173.0375) -> (-139.7, -169.8625) centre (-142.875, -169.8625) ccw
  arc A255 (-182.88, -167.3225) -> (-180.975, -173.0375) centre (-180.975, -169.8625) ccw
  line L264 (-133.35, 391.9093) -> (-133.35, 315.7093) construction
  line L265 (-127, -141.2875) -> (-127, -169.8625)
  arc A256 (-121.92, -138.7475) -> (-127, -141.2875) centre (-123.825, -141.2875) ccw
  arc A257 (-117.475, -119.0625) -> (-119.38, -124.7775) centre (-117.475, -122.2375) ccw
  line L266 (-76.2, -122.2375) -> (-76.2, -150.8125)
  arc A258 (-76.2, -122.2375) -> (-79.375, -119.0625) centre (-79.375, -122.2375) ccw
  line L267 (-117.475, -119.0625) -> (-79.375, -119.0625)
  arc A259 (-85.725, -173.0375) -> (-83.82, -167.3225) centre (-85.725, -169.8625) ccw
  line L268 (-81.28, -153.3525) -> (-119.38, -124.7775)
  line L269 (-83.82, -167.3225) -> (-121.92, -138.7475)
  line L270 (-123.825, -173.0375) -> (-85.725, -173.0375)
  arc A260 (-81.28, -153.3525) -> (-76.2, -150.8125) centre (-79.375, -150.8125) ccw
  arc A261 (-127, -169.8625) -> (-123.825, -173.0375) centre (-123.825, -169.8625) ccw
  line L271 (-190.5973, -179.3875) -> (-46.1334, -179.3875) construction
  line L272 (-127, -217.4875) -> (-127, -188.9125)
  arc A262 (-180.975, -185.7375) -> (-182.88, -191.4525) centre (-180.975, -188.9125) ccw
  line L273 (-142.875, -185.7375) -> (-180.975, -185.7375)
  arc A263 (-139.7, -188.9125) -> (-142.875, -185.7375) centre (-142.875, -188.9125) ccw
  line L274 (-190.5, -236.5375) -> (-190.5, -207.9625)
  line L275 (-182.88, -191.4525) -> (-144.78, -220.0275)
  line L276 (-139.7, -217.4875) -> (-139.7, -188.9125)
  line L277 (-185.42, -205.4225) -> (-147.32, -233.9975)
  arc A264 (-149.225, -239.7125) -> (-147.32, -233.9975) centre (-149.225, -236.5375) ccw
  line L278 (-149.225, -239.7125) -> (-187.325, -239.7125)
  arc A265 (-144.78, -220.0275) -> (-139.7, -217.4875) centre (-142.875, -217.4875) ccw
  line L279 (-76.2, -236.5375) -> (-76.2, -207.9625)
  arc A266 (-185.42, -205.4225) -> (-190.5, -207.9625) centre (-187.325, -207.9625) ccw
  arc A267 (-123.825, -185.7375) -> (-127, -188.9125) centre (-123.825, -188.9125) ccw
  arc A268 (-127, -217.4875) -> (-121.92, -220.0275) centre (-123.825, -217.4875) ccw
  arc A269 (-190.5, -236.5375) -> (-187.325, -239.7125) centre (-187.325, -236.5375) ccw
  line L280 (-123.825, -185.7375) -> (-85.725, -185.7375)
  line L281 (-83.82, -191.4525) -> (-121.92, -220.0275)
  arc A270 (-83.82, -191.4525) -> (-85.725, -185.7375) centre (-85.725, -188.9125) ccw
  arc A271 (-76.2, -207.9625) -> (-81.28, -205.4225) centre (-79.375, -207.9625) ccw
  arc A272 (-119.38, -233.9975) -> (-117.475, -239.7125) centre (-117.475, -236.5375) ccw
  line L282 (-117.475, -239.7125) -> (-79.375, -239.7125)
  arc A273 (-79.375, -239.7125) -> (-76.2, -236.5375) centre (-79.375, -236.5375) ccw
  line L283 (-81.28, -205.4225) -> (-119.38, -233.9975)
  line L284 (-63.5, -122.2375) -> (-63.5, -150.8125)
  arc A274 (-60.325, -119.0625) -> (-63.5, -122.2375) centre (-60.325, -122.2375) ccw
  line L285 (-58.42, -153.3525) -> (-20.32, -124.7775)
  line L286 (-22.225, -119.0625) -> (-60.325, -119.0625)
  arc A275 (-20.32, -124.7775) -> (-22.225, -119.0625) centre (-22.225, -122.2375) ccw
  arc A276 (-12.7, -141.2875) -> (-17.78, -138.7475) centre (-15.875, -141.2875) ccw
  line L287 (-55.88, -167.3225) -> (-17.78, -138.7475)
  line L288 (-12.7, -141.2875) -> (-12.7, -169.8625)
  line L289 (-15.875, -173.0375) -> (-53.975, -173.0375)
  arc A277 (-63.5, -150.8125) -> (-58.42, -153.3525) centre (-60.325, -150.8125) ccw
  arc A278 (-55.88, -167.3225) -> (-53.975, -173.0375) centre (-53.975, -169.8625) ccw
  arc A279 (-15.875, -173.0375) -> (-12.7, -169.8625) centre (-15.875, -169.8625) ccw
  arc A280 (47.625, -239.7125) -> (50.8, -236.5375) centre (47.625, -236.5375) ccw
  arc A281 (43.18, -191.4525) -> (41.275, -185.7375) centre (41.275, -188.9125) ccw
  arc A282 (3.175, -185.7375) -> (0, -188.9125) centre (3.175, -188.9125) ccw
  line L290 (-12.7, -217.4875) -> (-12.7, -188.9125)
  line L291 (-189.0098, -179.3875) -> (-44.5459, -179.3875) construction
  line L292 (0, -217.4875) -> (0, -188.9125)
  line L293 (3.175, -173.0375) -> (41.275, -173.0375)
  line L294 (3.175, -185.7375) -> (41.275, -185.7375)
  line L295 (43.18, -191.4525) -> (5.08, -220.0275)
  arc A283 (50.8, -207.9625) -> (45.72, -205.4225) centre (47.625, -207.9625) ccw
  line L296 (45.72, -205.4225) -> (7.62, -233.9975)
  line L297 (50.8, -236.5375) -> (50.8, -207.9625)
  line L298 (9.525, -239.7125) -> (47.625, -239.7125)
  arc A284 (5.08, -138.7475) -> (0, -141.2875) centre (3.175, -141.2875) ccw
  arc A285 (9.525, -119.0625) -> (7.62, -124.7775) centre (9.525, -122.2375) ccw
  line L299 (0, -141.2875) -> (0, -169.8625)
  line L300 (-6.35, 393.4968) -> (-6.35, 317.2968) construction
  arc A286 (41.275, -173.0375) -> (43.18, -167.3225) centre (41.275, -169.8625) ccw
  line L301 (43.18, -167.3225) -> (5.08, -138.7475)
  line L302 (9.525, -119.0625) -> (47.625, -119.0625)
  line L303 (45.72, -153.3525) -> (7.62, -124.7775)
  arc A287 (50.8, -122.2375) -> (47.625, -119.0625) centre (47.625, -122.2375) ccw
  line L304 (50.8, -122.2375) -> (50.8, -150.8125)
  arc A288 (45.72, -153.3525) -> (50.8, -150.8125) centre (47.625, -150.8125) ccw
  arc A289 (0, -169.8625) -> (3.175, -173.0375) centre (3.175, -169.8625) ccw
  arc A290 (-12.7, -188.9125) -> (-15.875, -185.7375) centre (-15.875, -188.9125) ccw
  arc A291 (0, -217.4875) -> (5.08, -220.0275) centre (3.175, -217.4875) ccw
  arc A292 (7.62, -233.9975) -> (9.525, -239.7125) centre (9.525, -236.5375) ccw
  arc A293 (-17.78, -220.0275) -> (-12.7, -217.4875) centre (-15.875, -217.4875) ccw
  arc A294 (-63.5, -236.5375) -> (-60.325, -239.7125) centre (-60.325, -236.5375) ccw
  line L305 (-63.5, -236.5375) -> (-63.5, -207.9625)
  line L306 (-22.225, -239.7125) -> (-60.325, -239.7125)
  arc A295 (-58.42, -205.4225) -> (-63.5, -207.9625) centre (-60.325, -207.9625) ccw
  arc A296 (-22.225, -239.7125) -> (-20.32, -233.9975) centre (-22.225, -236.5375) ccw
  arc A297 (-53.975, -185.7375) -> (-55.88, -191.4525) centre (-53.975, -188.9125) ccw
  line L307 (-58.42, -205.4225) -> (-20.32, -233.9975)
  line L308 (-55.88, -191.4525) -> (-17.78, -220.0275)
  line L309 (-15.875, -185.7375) -> (-53.975, -185.7375)
  arc A298 (66.675, -119.0625) -> (63.5, -122.2375) centre (66.675, -122.2375) ccw
  line L310 (104.775, -119.0625) -> (66.675, -119.0625)
  line L311 (127, -141.2875) -> (127, -169.8625)